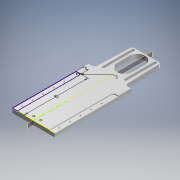
# Autodesk Inventor part: Z-baseplate
Saved by Autodesk Inventor 2016 (Build 200138000, 138)
## iProperties
Created: 2015-04-22
Part Number: Z-baseplate
Material: Aluminum 6061
Document SubType Name: Modeling
Designer: ax
Density: 2.7 g/cm^3
Appearance: Aluminum - Flat
Mass: 117.71 g
Surface Area: 198.204 cm^2
Volume: 43.5963 cm^3
Author: ax
Autodesk Inventor part; units mm, degrees
ref_plane "YZ Plane" through (0, 0, 0) normal (1, 0, 0) x (0, 1, 0)
ref_plane "XZ Plane" through (0, 0, 0) normal (0, 1, 0) x (-1, 0, 0)
ref_plane "XY Plane" through (0, 0, 0) normal (0, 0, 1) x (1, 0, 0)
sketch "Sketch1" plane through (0, 0, 0) normal (0, 0, 1) x (1, 0, 0)
  line L0 (0, 0) -> (60, 0)
  line L1 (60, 0) -> (60, 160)
  line L2 (60, 160) -> (0, 160)
  line L3 (0, 160) -> (0, 0)
  dimension "d0" = 60
  dimension "d1" = 160
  constraints: 8 end point, 2 parallel, 1 horizontal, 1 perpendicular
  measures "d0" distance of L2.end L1.end
  measures "d1" distance of L1.end L0.end
extrude "Extrusion1" add sketch "Sketch1" along normal blind 6
sketch "Sketch2" plane through (0, 0, 6) normal (0, 0, 1) x (1, 0, 0)
  line L0 (30, 170) -> (30, -10) construction
  line L1 (14.5, 170) -> (14.5, -10) construction
  line L2 (30, 158) -> (30, 118) construction
  line L3 (18.975, 146.975) -> (18.975, 129.025)
  line L4 (41.025, 129.025) -> (41.025, 146.975)
  arc A0 (41.025, 146.975) -> (18.975, 146.975) centre (30, 146.975) ccw
  arc A1 (18.975, 129.025) -> (41.025, 129.025) centre (30, 129.025) ccw
  line L5 (14.5, 158) -> (14.5, 113) construction
  line L6 (12.75, 156.25) -> (12.75, 114.75)
  line L7 (16.25, 114.75) -> (16.25, 156.25)
  arc A2 (16.25, 156.25) -> (12.75, 156.25) centre (14.5, 156.25) ccw
  arc A3 (12.75, 114.75) -> (16.25, 114.75) centre (14.5, 114.75) ccw
  line L8 (45.5, 158) -> (45.5, 113) construction
  line L9 (47.25, 156.25) -> (47.25, 114.75)
  line L10 (43.75, 114.75) -> (43.75, 156.25)
  arc A4 (47.25, 156.25) -> (43.75, 156.25) centre (45.5, 156.25) ccw
  arc A5 (43.75, 114.75) -> (47.25, 114.75) centre (45.5, 114.75) ccw
  point P0 (0, 0)
  point P1 (30, 138)
  point P2 (14.5, 135.5)
  point P3 (45.5, 135.5)
  dimension "d5" = 15.5
  dimension "d6" = 40
  dimension "d7" = 22.05
  dimension "d8" = 45
  dimension "d9" = 3.5
  constraints: 28 end point, 18 point on circle, 9 point on line, 9 symmetric about line, 8 tangent, 6 centre point, 3 parallel, 2 midpoint, 1 vertical, 2 other
  measures "d5" distance between parallel lines of L0 L1
  measures "d6" distance of L2.start L2.end
  measures "d7" diameter of A1
  measures "d8" distance of L5.start L5.end
  measures "d9" diameter of A3
extrude "Extrusion2" cut sketch "Sketch2" against normal through all
sketch "Sketch3" plane through (0, 0, 6) normal (0, 0, 1) x (1, 0, 0)
  line L0 (60, 160) -> (0, 160) projected
  line L1 (30, 160) -> (30, 60)
  line L2 (10, 160) -> (8.1852, 108.0317)
  line L3 (10, 160) -> (62, 160) construction
  line L4 (8.1852, 108.0317) -> (0, 108.0317)
  line L5 (0, 160) -> (0, 0) projected
  line L6 (10, 160) -> (0, 160)
  line L7 (0, 160) -> (0, 108.0317)
  line L8 (50, 160) -> (51.8148, 108.0317)
  line L9 (51.8148, 108.0317) -> (60, 108.0317)
  line L10 (50, 160) -> (60, 160)
  line L11 (60, 160) -> (60, 108.0317)
  dimension "d12" = 100
  dimension "d13" = 52
  dimension "d14" = 92
  dimension "d15" = 92
  constraints: 20 end point, 3 symmetric about line, 2 collinear, 2 point on line, 1 equal length, 1 horizontal, 1 midpoint, 1 vertical
  measures "d12" distance of L1.start L1.end
  measures "d13" distance of L2.start L2.end
  measures "d14" angle of L2 L3
  measures "d15" angle of L2 L4
extrude "Extrusion3" cut sketch "Sketch3" against normal through all
fillet "Fillet1" radius 3 4 edges at (51.8148, 108.0317, 3) (50, 160, 3) (10, 160, 3) (8.1852, 108.0317, 3)
sketch "Sketch4" plane through (0, 0, 6) normal (0, 0, 1) x (1, 0, 0)
  line L0 (30, 0) -> (30, 50)
  line L1 (0, 0) -> (60, 0) projected
  line L2 (0, 0) -> (7, 0)
  line L3 (7, 0) -> (7, 87)
  line L4 (4, 90) -> (0, 90)
  line L5 (0, 90) -> (0, 0)
  arc A0 (7, 87) -> (4, 90) centre (4, 87) ccw
  point P0 (25, 5)
  point P1 (35, 5)
  point P2 (7, 90)
  dimension "d27" = 7
  dimension "d28" = 90
  dimension "d29" = 3
  constraints: 10 end point, 2 parallel, 2 point on circle, 2 point on line, 2 tangent, 1 centre point, 1 horizontal, 1 perpendicular, 1 symmetric about line, 1 vertical
  measures "d27" distance of L4.end point (7, 90)
  measures "d28" distance of point (7, 90) L2.end
  measures "d29" radius of A0
hole "Hole1" at (25, 5, 6) at (35, 5, 6) direction (0, 0, -1) diameter 4 end through all
extrude "Extrusion4" cut sketch "Sketch4" against normal blind 1.2
sketch "Sketch6" plane through (0, 0, 4.8) normal (0, 0, 1) x (1, 0, 0)
  line L0 (7, 0) -> (0, 0) projected
  line L1 (0, 108.0317) -> (0, 0) projected
  point P0 (3.5, 10)
  point P1 (3.5, 25)
  point P2 (3.5, 40)
  point P3 (3.5, 55)
  point P4 (3.5, 70)
  dimension "d32" = 10
  dimension "d33" = 3.5
  dimension "d36" = 15
  constraints: 1 vertical, 4 other
  measures "d32" distance from line of L0 point (3.5, 10)
  measures "d33" distance from line of L1 point (3.5, 10)
  measures "d36" distance of point (3.5, 10) point (3.5, 25)
hole "Hole2" at (3.5, 10, 4.8) at (3.5, 25, 4.8) at (3.5, 40, 4.8) at (3.5, 55, 4.8) at (3.5, 70, 4.8) direction (0, 0, -1) diameter 2 end through all
ref_plane "Work Plane1" through (30, 0, 6) normal (1, 0, 0) x (0, 1, 0)
mirror "Mirror1" about plane through (30, 0, 6) normal (1, 0, 0) of "Extrusion4", "Hole2"
ref_plane "Work Plane2" through (30, 0, 6) normal (1, 0, 0) x (0, 1, 0)
body "Solid1"
